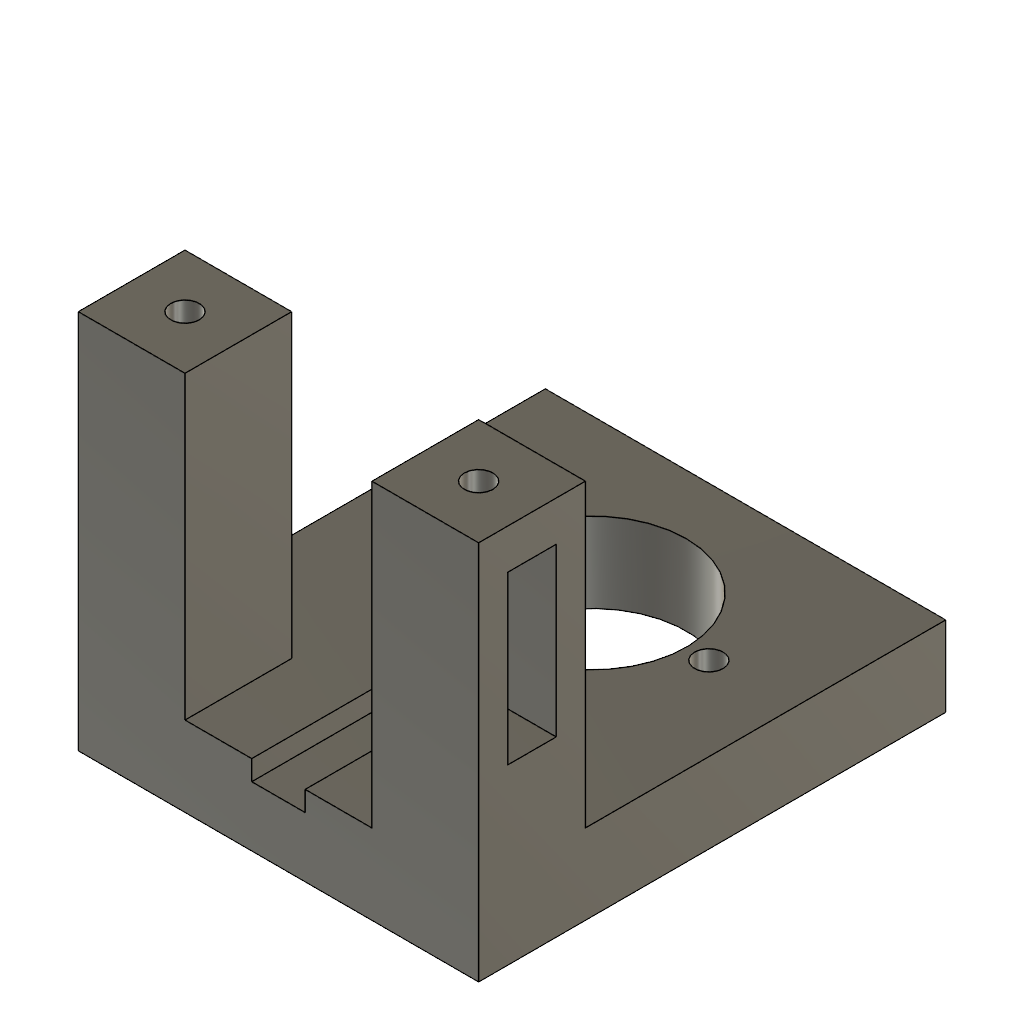
04 - PRIMARY SUPPORT MECHANISM ( RIGHT SIDE ) (Autodesk Fusion 360 design; units mm, degrees)
Autodesk Fusion 360 part; units mm, degrees
sketch "01 - PRIMARY SUPPORT MECHANISM ( RIGHT SIDE ) SKETCH" plane through (0, 0, 0) normal (0, 0, 1) x (1, 0, 0)
  line L0 (-30, 35) -> (30, 35)
  line L1 (30, 35) -> (30, -35)
  line L2 (30, -35) -> (-30, -35)
  line L3 (-30, -35) -> (-30, 35)
  line L4 (-30, -19) -> (30, -19) construction
  line L5 (0, -35) -> (0, -5.422) construction
  line L6 (7.6, -5.422) -> (7.6, 0.1231)
  arc A0 (7.6, 0.1231) -> (-7.6, 0.1231) centre (0, 11.9996) ccw
  line L7 (-7.6, -5.422) -> (7.6, -5.422)
  line L8 (-7.6, -5.422) -> (-7.6, 0.1231)
  line L9 (4, -5.422) -> (4, -35)
  line L10 (-4, -5.422) -> (-4, -35)
  line L11 (-17.5, 11.9996) -> (17.5, 11.9996) construction
  circle A1 centre (17.5, 11.9996) radius 2.14
  line L12 (21.125, 14.0925) -> (17.5, 16.1854)
  line L13 (17.5, 16.1854) -> (13.875, 14.0925)
  line L14 (13.875, 14.0925) -> (13.875, 9.9067)
  line L15 (13.875, 9.9067) -> (17.5, 7.8138)
  line L16 (17.5, 7.8138) -> (21.125, 9.9067)
  line L17 (21.125, 9.9067) -> (21.125, 14.0925)
  line L18 (17.5, 11.9996) -> (17.5, 14.1396) construction
  circle A2 centre (-17.5, 11.9996) radius 2.14
  line L19 (-13.875, 9.9067) -> (-13.875, 14.0925)
  line L20 (-13.875, 14.0925) -> (-17.5, 16.1854)
  line L21 (-17.5, 16.1854) -> (-21.125, 14.0925)
  line L22 (-21.125, 14.0925) -> (-21.125, 9.9067)
  line L23 (-21.125, 9.9067) -> (-17.5, 7.8138)
  line L24 (-17.5, 7.8138) -> (-13.875, 9.9067)
  line L25 (-17.5, 11.9996) -> (-17.5, 14.1396) construction
  point P0 (17.5, 11.9996)
  point P1 (-17.5, 11.9996)
  dimension "d1" = 60
  dimension "d2" = 70
  dimension "d3" = 30
  dimension "d4" = 35
  dimension "d5" = 16
  dimension "d12" = 29.578
  dimension "d14" = 15.2
  dimension "d15" = 5.5451
  dimension "d16" = 14.1
  dimension "d21" = 17.4216
  dimension "d24" = 8
  dimension "d25" = 4
  dimension "d55" = 35
  dimension "d56" = 4.28
  dimension "d57" = 3.625
  dimension "d58" = 4.28
  dimension "d59" = 3.625
  constraint horizontal L0
  constraint vertical L1
  constraint horizontal L2
  constraint vertical L3
  constraint coincident L3 L4.start
  constraint coincident L1 L4.end
  constraint perpendicular L1 L4
  constraint midpoint L2 L5.start
  constraint perpendicular L4 L5
  constraint equal L6 L8
  constraint parallel L6 L8
  constraint perpendicular L6 L7
  constraint coincident L5.end L7
  constraint midpoint L5.end L7
  constraint horizontal L7
  constraint coincident L7 L9.start
  constraint coincident L2 L9.end
  constraint perpendicular L2 L9
  constraint coincident L7 L10.start
  constraint coincident L2 L10.end
  constraint perpendicular L2 L10
  constraint horizontal L11
  constraint midpoint A0.centre L11
  constraint coincident P0 L11.end
  constraint coincident A1 L18.end
  constraint perpendicular L11 L18
  constraint coincident L12.end L18
  constraint coincident P1 L11.start
  constraint coincident A2 L25.end
  constraint perpendicular L11 L25
  constraint coincident L20.end L25
  measures "d1" distance of L0.start L0.end
  measures "d2" distance of L0.start L2.end
  measures "d3" distance of origin L3
  measures "d4" distance of origin L0
  measures "d5" distance of L2 L4
  measures "d12" distance of L5.start L5.end
  measures "d14" distance of L7.start L6.start
  measures "d15" distance of L6.end L6.start
  measures "d16" radius of A0
  measures "d21" distance of A0.centre L7
  measures "d24" distance of L9 L10
  measures "d25" distance of L5 L10
  measures "d55" horizontal distance of P1 P0
  measures "d56" diameter of A1
  measures "d57" distance of P0 L17
  measures "d58" diameter of A2
  measures "d59" distance of P1 L24
extrude "Extrude2" add sketch "01 - PRIMARY SUPPORT MECHANISM ( RIGHT SIDE ) SKETCH" along normal blind 12 contours L0 L1 L2 L3 L6 A0 L7 L8 L9 L10 L12 L13 L15 L16 L17 L20 L21 L22 L23 L24 | A0 L20 L21 L22 L23 L24 | A0 L12 L13 L15 L16 L17 | A1 | A2
extrude "Extrude3" add sketch "01 - PRIMARY SUPPORT MECHANISM ( RIGHT SIDE ) SKETCH" along normal blind 9 contours L2 L7 L9 L10
sketch "02 - PRIMARY SUPPORT MECHANISM ( RIGHT SIDE ) SKETCH" plane through (0, 0, 12) normal (0, 0, 1) x (-1, 0, 0)
  line L0 (7.6, 5.422) -> (7.6, -0.1231)
  arc A0 (-7.6, -0.1231) -> (7.6, -0.1231) centre (0, -11.9996) ccw
  line L1 (-7.6, -0.1231) -> (-7.6, 5.422)
  line L2 (-7.6, 5.422) -> (-4, 5.422)
  line L3 (-4, 5.422) -> (-4, 35)
  line L4 (-4, 35) -> (-30, 35)
  line L5 (-30, 35) -> (-30, -35)
  line L6 (-30, -35) -> (30, -35)
  line L7 (30, -35) -> (30, 35)
  line L8 (30, 35) -> (4, 35)
  line L9 (4, 35) -> (4, 5.422)
  line L10 (4, 5.422) -> (7.6, 5.422)
  line L11 (30, 35) -> (14, 35)
  line L12 (14, 35) -> (14, 19)
  line L13 (14, 19) -> (30, 19)
  line L14 (30, 19) -> (30, 35)
  line L15 (-30, 35) -> (-14, 35)
  line L16 (-14, 35) -> (-14, 19)
  line L17 (-14, 19) -> (-30, 19)
  line L18 (-30, 19) -> (-30, 35)
  dimension "d30" = 16
  dimension "d31" = 16
  dimension "d32" = 16
  dimension "d33" = 16
  constraint horizontal L11
  constraint vertical L12
  constraint horizontal L13
  constraint vertical L14
  constraint coincident L7.end L8.start
  constraint horizontal L15
  constraint vertical L16
  constraint horizontal L17
  constraint vertical L18
  constraint coincident L4.end L5.start
  measures "d30" distance of L7.end L11.end
  measures "d31" distance of L7.end L13.end
  measures "d32" distance of L4.end L15.end
  measures "d33" distance of L4.end L17.end
extrude "Extrude4" add sketch "02 - PRIMARY SUPPORT MECHANISM ( RIGHT SIDE ) SKETCH" along normal blind 45 contours L7 L8 L11 L12 L13 L14 | L4 L5 L15 L16 L17 L18
sketch "03 - PRIMARY SUPPORT MECHANISM ( RIGHT SIDE ) SKETCH" plane through (0, 0, 57) normal (0, 0, 1) x (-1, 0, 0)
  line L0 (-30, 19) -> (-14, 19)
  line L1 (-14, 19) -> (-14, 35)
  line L2 (-14, 35) -> (-30, 35)
  line L3 (-30, 35) -> (-30, 19)
  line L4 (-14, 27) -> (-30, 27) construction
  line L5 (-22, 19) -> (-22, 35) construction
  line L6 (-25.625, 24.9071) -> (-22, 22.8142)
  line L7 (-22, 22.8142) -> (-18.375, 24.9071)
  line L8 (-18.375, 24.9071) -> (-18.375, 29.0929)
  line L9 (-18.375, 29.0929) -> (-22, 31.1858)
  line L10 (-22, 31.1858) -> (-25.625, 29.0929)
  line L11 (-25.625, 29.0929) -> (-25.625, 24.9071)
  line L12 (-22, 22.8142) -> (-30, 22.8142)
  line L13 (-22, 31.1858) -> (-30, 31.1858)
  line L14 (-30, 31.1858) -> (-30, 22.8142)
  circle A0 centre (-22, 27) radius 3.625
  line L15 (-22, 23.375) -> (-22, 22.8142)
  line L16 (-22, 31.1858) -> (-22, 30.625)
  line L17 (-22, 23.375) -> (-30, 23.375)
  line L18 (-22, 30.625) -> (-30, 30.625)
  circle A1 centre (-22, 27) radius 2.14
  point P0 (-22, 27)
  dimension "d36" = 3.625
  dimension "d42" = 4.28
  constraint midpoint L1 L4.start
  constraint midpoint L3 L4.end
  constraint midpoint L0 L5.start
  constraint midpoint L2 L5.end
  constraint midpoint L4 P0
  constraint coincident L5 L9.end
  constraint coincident L3 L12.end
  constraint perpendicular L3 L12
  constraint coincident L3 L13.end
  constraint perpendicular L3 L13
  constraint coincident P0 A0.centre
  constraint tangent L11 A0
  constraint coincident A0 L15.start
  constraint coincident L5 L15.start
  constraint coincident A0 L16.end
  constraint coincident L5 L16.end
  constraint coincident L14 L17.end
  constraint tangent A0 L17
  constraint coincident L14 L18.end
  constraint tangent A0 L18
  measures "d36" distance of P0 L11
  measures "d42" diameter of A1
extrude "Extrude5" cut sketch "03 - PRIMARY SUPPORT MECHANISM ( RIGHT SIDE ) SKETCH" against normal blind 25 from surface at -6 contours L3 L6 L10 L11 L14 L17 L18 | L6 A0 L17 | A0 | L10 A0 L18 | L6 L11 A0 | L10 L11 A0 | A1
extrude "Extrude7" cut sketch "03 - PRIMARY SUPPORT MECHANISM ( RIGHT SIDE ) SKETCH" against normal blind 6 contours A1
sketch "04 - PRIMARY SUPPORT MECHANISM ( RIGHT SIDE ) SKETCH" plane through (0, 0, 57) normal (0, 0, 1) x (-1, 0, 0)
  line L0 (30, 19) -> (30, 35)
  line L1 (30, 35) -> (14, 35)
  line L2 (14, 35) -> (14, 19)
  line L3 (14, 19) -> (30, 19)
  line L4 (30, 27) -> (14, 27) construction
  line L5 (22, 35) -> (22, 19) construction
  line L6 (18.375, 24.9071) -> (22, 22.8142)
  line L7 (22, 22.8142) -> (25.625, 24.9071)
  line L8 (25.625, 24.9071) -> (25.625, 29.0929)
  line L9 (25.625, 29.0929) -> (22, 31.1858)
  line L10 (22, 31.1858) -> (18.375, 29.0929)
  line L11 (18.375, 29.0929) -> (18.375, 24.9071)
  circle A0 centre (22, 27) radius 3.625
  circle A1 centre (22, 27) radius 2.14
  line L12 (22, 22.8142) -> (30, 22.8142)
  line L13 (22, 31.1858) -> (30, 31.1858)
  line L14 (30, 31.1858) -> (30, 22.8142)
  line L15 (22, 23.375) -> (30, 23.375)
  line L16 (22, 30.625) -> (30, 30.625)
  point P0 (22, 27)
  dimension "d45" = 3.625
  dimension "d46" = 4.28
  constraint midpoint L0 L4.start
  constraint midpoint L2 L4.end
  constraint midpoint L1 L5.start
  constraint midpoint L3 L5.end
  constraint midpoint L5 P0
  constraint coincident L5 L9.end
  constraint coincident P0 A0.centre
  constraint tangent L11 A0
  constraint coincident L0 L12.end
  constraint perpendicular L0 L12
  constraint coincident L0 L13.end
  constraint perpendicular L0 L13
  constraint coincident A0 L15.start
  constraint coincident L5 L15.start
  constraint coincident L14 L15.end
  constraint coincident A0 L16.start
  constraint coincident L5 L16.start
  constraint coincident L14 L16.end
  constraint tangent A0 L15
  constraint tangent A0 L16
  measures "d45" distance of P0 L11
  measures "d46" diameter of A1
extrude "Extrude9" cut sketch "04 - PRIMARY SUPPORT MECHANISM ( RIGHT SIDE ) SKETCH" against normal blind 25 from surface at -6 contours L0 L7 L8 L9 L14 L15 L16 | L7 A0 L15 | A0 | L9 A0 L16 | L7 L8 A0 | L8 L9 A0 | A1
extrude "Extrude10" cut sketch "04 - PRIMARY SUPPORT MECHANISM ( RIGHT SIDE ) SKETCH" against normal blind 6 contours A1
extrude "Extrude11" cut sketch "01 - PRIMARY SUPPORT MECHANISM ( RIGHT SIDE ) SKETCH" along normal blind 12 contours A1 | A2
extrude "Extrude12" cut sketch "01 - PRIMARY SUPPORT MECHANISM ( RIGHT SIDE ) SKETCH" along normal blind 4 contours A0 L20 L21 L22 L23 L24 | A0 L12 L13 L15 L16 L17
named bodies: "01 - PRIMARY SUPPORT MECHANISM ( RIGHT SIDE )"
